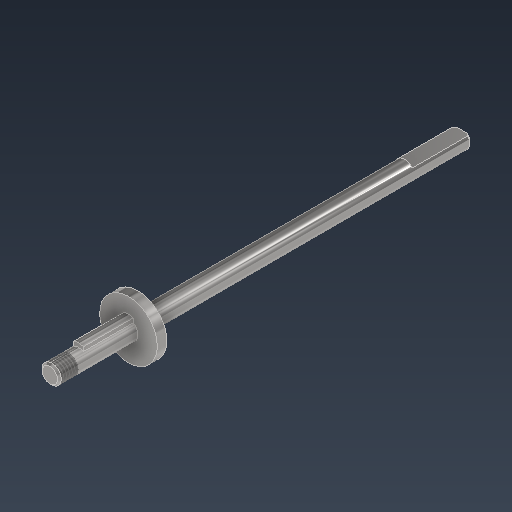
# Autodesk Inventor part: ballInletWheelAxle
Saved by Autodesk Inventor 2021.4 (Build 254397000, 397)
## iProperties
Created: 2022-03-02
Part Number: ballInletWheelAxle
Material: Generic
Document SubType Name: Modeling
Designer: jo_ki
Density: 1 g/cm^3
Appearance: Steel - Polished
Author: jo_ki
Autodesk Inventor part; units mm, degrees
ref_plane "YZ Plane" through (0, 0, 0) normal (1, 0, 0) x (0, 1, 0)
ref_plane "XZ Plane" through (0, 0, 0) normal (0, 1, 0) x (-1, 0, 0)
ref_plane "XY Plane" through (0, 0, 0) normal (0, 0, 1) x (1, 0, 0)
derived "Mastersketch.ipt"
sketch "Sketch1" plane through (0, 0, 0) normal (1, 0, 0) x (0, 1, 0)
  line L0 (5, -10) -> (-5, -10)
  line L1 (-5, -10) -> (-5, -41)
  line L2 (-5, -41) -> (5, -41)
  line L3 (5, -41) -> (5, -10)
  line L4 (15, -41) -> (-15, -41)
  line L5 (-15, -41) -> (-15, -46)
  line L6 (-15, -46) -> (15, -46)
  line L7 (15, -46) -> (15, -41)
  line L8 (5, -46) -> (-5, -46)
  line L9 (-5, -46) -> (-5, -219.8)
  line L10 (-5, -219.8) -> (5, -219.8)
  line L11 (5, -219.8) -> (5, -46)
  line L12 (0, -263.76) -> (0, 43.96) projected
  line L13 (5, -10) -> (-5, -10)
  line L14 (-5, -10) -> (-5, 0)
  line L15 (-5, 0) -> (5, 0)
  line L16 (5, 0) -> (5, -10)
  line L17 (-21, 0) -> (21, 0) projected
  line L18 (5, -219.8) -> (-5, -219.8)
  line L19 (-5, -219.8) -> (-5, -214.8)
  line L20 (-5, -214.8) -> (5, -214.8)
  line L21 (5, -214.8) -> (5, -219.8)
  point P0 (0, 0)
  point P1 (0, 0)
  point P2 (0, -214.8)
  dimension "d0" = 10
  dimension "d1" = 31
  dimension "d3" = 10
  dimension "d7" = 5
  dimension "d8" = 10
  dimension "d9" = 178.8
  dimension "d10" = 5
  constraints: 40 end point, 10 parallel, 5 horizontal, 5 perpendicular, 3 collinear, 3 point on line, 3 other
  measures "d0" distance between parallel lines of L1 L3
  measures "d1" distance between parallel lines of L0 L2
  measures "d3" distance between parallel lines of L15 L0
  measures "d7" distance of L6.end L4.start
  measures "d8" distance between parallel lines of L3 L7
  measures "d9" distance between parallel lines of L2 L10
  measures "d10" distance between parallel lines of L20 L10
revolve "Revolution1" add sketch "Sketch1" angle 360 about axis through (0, 0, -10) along (0, 0, 1) contours L3 L2 L12 L0 | L0 L12 L15 L16 | L4 L7 L6 L12 L2 | L6 L11 L20 L12
thread "Thread2" size "M10x1.5" class "6g" standard "ANSI Metric M Profile" length 10
chamfer "Chamfer1" distance 1 angle 45 2 edges at (0, -5, 0) (0, -5, -214.8)
sketch "Sketch2" plane through (0, 0, -214.8) normal (0, 0, -1) x (-1, 0, 0)
  circle A0 centre (0, 0) radius 5 projected
  circle A1 centre (0, 0) radius 5 projected
  line L0 (-4, 3) -> (4, 3)
  dimension "d21" = 2
  constraints: 2 end point, 2 point on circle, 1 horizontal
  measures "d21" distance edge to line of A0 L0
extrude "Extrusion2" cut sketch "Sketch2" against normal blind 30 contours L0 A0 picked at (1.0679, 3.2796)
sketch "Sketch3" plane through (0, 0, -41) normal (0, 0, 1) x (1, 0, 0)
  circle A0 centre (0, 0) radius 5 projected
  line L0 (-2.5, 7) -> (2.5, 7)
  line L1 (2.5, 7) -> (2.5, 0)
  line L2 (2.5, 0) -> (-2.5, 0)
  line L3 (-2.5, 0) -> (-2.5, 7)
  circle A1 centre (0, 0) radius 7
  line L4 (0, -21) -> (0, 21) projected
  point P0 (-2.5, 6.5383)
  point P1 (-2.5, 4.3301)
  point P2 (2.5, 4.3301)
  point P3 (2.5, 6.5383)
  dimension "d46" = 5
  dimension "d47" = 2
  constraints: 8 end point, 2 parallel, 1 centre point, 1 coincident, 1 horizontal, 1 midpoint, 1 perpendicular, 1 tangent, 1 other
  measures "d46" distance between parallel lines of L3 L1
  measures "d47" distance edge to line of A0 L0
extrude "Extrusion3" add sketch "Sketch3" along normal blind 26 contours A0 L4 A1 L1 | A0 L3 A1 L4 picked at (1.422, 5.472) picked at (-1.422, 5.472)
equation "\"d0\" = ballInletWheelDriveShaftAxle_diameter"
equation "\"d1\" = ballInletWheel_thickness"
equation "\"ballInletWheelDriveShaftAxle_diameter\" = 10"
equation "\"ballInletWheel_thickness\" = 31"
body "Solid1"
